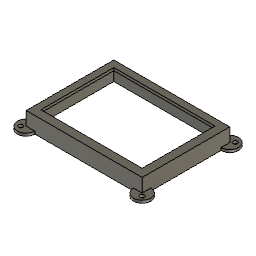
StepperBreadboardHolder (Autodesk Fusion 360 design; units mm, degrees)
part number: 2026-05-25-11-22-07-482
Autodesk Fusion 360 part; units mm, degrees
sketch "Sketch1" plane through (0, 0, 0) normal (0, 0, 1) x (1, 0, 0)
  line L0 (0, 0) -> (82, 0)
  line L1 (82, 0) -> (82, 61)
  line L2 (82, 61) -> (0, 61)
  line L3 (0, 61) -> (0, 0)
  line L4 (-2, 63) -> (84, 63)
  line L5 (84, 63) -> (84, -2)
  line L6 (84, -2) -> (-2, -2)
  line L7 (-2, -2) -> (-2, 63)
  circle A0 centre (-2, -2) radius 6.5
  circle A1 centre (-2, 63) radius 6.5
  circle A2 centre (84, 63) radius 6.5
  circle A3 centre (84, -2) radius 6.5
  circle A4 centre (-4, -4) radius 1.65
  circle A5 centre (-4, 65) radius 1.65
  circle A6 centre (86, 65) radius 1.65
  circle A7 centre (86, -4) radius 1.65
  line L8 (3, 58) -> (78, 58)
  line L9 (78, 58) -> (78, 4)
  line L10 (78, 4) -> (3, 4)
  line L11 (3, 4) -> (3, 58)
  dimension "d1" = 61
  dimension "d2" = 82
  dimension "d3" = 2
  dimension "d4" = 2
  dimension "d5" = 2
  dimension "d6" = 2
  dimension "d7" = 13
  dimension "d8" = 13
  dimension "d9" = 13
  dimension "d10" = 13
  dimension "d11" = 3.3
  dimension "d12" = 2
  dimension "d13" = 2
  dimension "d14" = 3.3
  dimension "d15" = 2
  dimension "d16" = 2
  dimension "d17" = 3.3
  dimension "d18" = 2
  dimension "d19" = 2
  dimension "d20" = 3.3
  dimension "d21" = 2
  dimension "d22" = 2
  dimension "d23" = 3
  dimension "d24" = 4
  dimension "d25" = 3
  dimension "d26" = 4
  constraint horizontal L0
  constraint vertical L1
  constraint horizontal L2
  constraint vertical L3
  constraint coincident L0.start L3.end
  constraint horizontal L4
  constraint vertical L5
  constraint horizontal L6
  constraint vertical L7
  constraint coincident L6.end L7.start
  constraint coincident L4.start L7.end
  constraint coincident L4.end L5.start
  constraint coincident L5.end L6.start
  constraint horizontal L8
  constraint vertical L9
  constraint horizontal L10
  constraint vertical L11
  measures "d1" distance of L0.start L2.end
  measures "d2" distance of L0.start L0.end
  measures "d3" distance of L2 L4
  measures "d4" distance of L1 L5
  measures "d5" distance of L3 L7
  measures "d6" distance of L0 L6
  measures "d7" diameter of A0
  measures "d8" diameter of A1
  measures "d9" diameter of A2
  measures "d10" diameter of A3
  measures "d11" diameter of A4
  measures "d12" vertical distance of L6.end A4.centre
  measures "d13" horizontal distance of L6.end A4.centre
  measures "d14" diameter of A5
  measures "d15" vertical distance of L4.start A5.centre
  measures "d16" horizontal distance of L4.start A5.centre
  measures "d17" diameter of A6
  measures "d18" horizontal distance of L4.end A6.centre
  measures "d19" vertical distance of L4.end A6.centre
  measures "d20" diameter of A7
  measures "d21" horizontal distance of L5.end A7.centre
  measures "d22" vertical distance of L5.end A7.centre
  measures "d23" distance of L2 L8
  measures "d24" distance of L0 L10
  measures "d25" distance of L3 L11
  measures "d26" distance of L1 L9
extrude "Extrude1" add sketch "Sketch1" along normal blind 2 contours L6 L7 A0 | L5 L6 A3 | L4 L7 A1 | L4 L5 A2 makes body 1 at (85.5519, 61.1596, 2) makes body 2 at (85.5519, -0.1596, 0) makes body 3 at (-3.5519, 61.1596, 0) makes body 4 at (-3.5519, -0.1596, 0)
extrude "Extrude2" add sketch "Sketch1" along normal blind 10 contours L0 L3 L6 L7 A0 | L0 L6 A0 A3 | L3 L7 A0 A1 | L0 L1 L5 L6 A3 | L2 L3 L4 L7 A1 | L1 L5 A2 A3 | L2 L4 A1 A2 | L1 L2 L4 L5 A2 bodies 1 2 3 4
extrude "Extrude3" add sketch "Sketch1" along normal blind 2 from surface at 10 contours L0 L3 A0 | L0 L3 L6 L7 A0 | L0 L1 L2 L3 A0 A1 A2 A3 | L0 L6 A0 A3 | L3 L7 A0 A1 | L0 L1 A3 | L0 L1 L5 L6 A3 | L2 L3 L4 L7 A1 | L2 L3 A1 | L1 L5 A2 A3 | L2 L4 A1 A2 | L1 L2 A2 | L1 L2 L4 L5 A2 bodies 1
